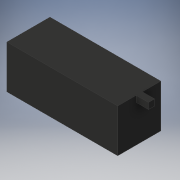
# Autodesk Inventor part: batery
Saved by Autodesk Inventor 2017 (Build 210142000, 142)
## iProperties
Created: 2017-10-06
Part Number: batery
Material: Rubber
Document SubType Name: Modeling
Designer: User
Density: 0.93 g/cm^3
Appearance: Rubber - Black
Author: User
Autodesk Inventor part; units mm, degrees
ref_plane "YZ Plane" through (0, 0, 0) normal (1, 0, 0) x (0, 1, 0)
ref_plane "XZ Plane" through (0, 0, 0) normal (0, 1, 0) x (-1, 0, 0)
ref_plane "XY Plane" through (0, 0, 0) normal (0, 0, 1) x (1, 0, 0)
sketch "Sketch1" plane through (0, 0, 0) normal (0, 0, 1) x (1, 0, 0)
  line L0 (0, 0) -> (114.3, 0)
  line L1 (114.3, 0) -> (114.3, 44.45)
  line L2 (114.3, 44.45) -> (0, 44.45)
  line L3 (0, 44.45) -> (0, 0)
  dimension "d0" = 114.3
  dimension "d1" = 44.45
  constraints: 8 end point, 2 parallel, 1 horizontal, 1 perpendicular
  measures "d0" distance of L2.end L1.end
  measures "d1" distance of L1.end L0.end
extrude "Extrusion1" add sketch "Sketch1" along normal blind 44.45
sketch "Sketch2" plane through (114.3, 0, 0) normal (1, 0, 0) x (0, 0, -1)
  line L0 (0, 44.45) -> (-44.45, 44.45) projected
  line L1 (-25.4, 44.45) -> (-19.05, 44.45)
  line L2 (-19.05, 44.45) -> (-19.05, 38.1)
  line L3 (-19.05, 38.1) -> (-25.4, 38.1)
  line L4 (-25.4, 38.1) -> (-25.4, 44.45)
  line L5 (-44.45, 0) -> (-44.45, 44.45) projected
  line L6 (0, 0) -> (0, 44.45) projected
  dimension "d4" = 19.05
  dimension "d5" = 19.05
  dimension "d6" = 6.35
  dimension "d7" = 6.35
  constraints: 8 end point, 2 parallel, 1 horizontal, 1 perpendicular, 1 point on line
  measures "d4" distance between parallel lines of L4 L5
  measures "d5" distance between parallel lines of L6 L2
  measures "d6" distance between parallel lines of L2 L4
  measures "d7" distance between parallel lines of L3 L0
extrude "Extrusion2" add sketch "Sketch2" along normal blind 12.7
body "Solid1"
